Links  big screw_v1 (Autodesk Fusion 360 design; units mm, degrees)
Autodesk Fusion 360 part; units mm, degrees
note: some values were not read from the file. Chosen so that the rebuilt part matches the saved one: which bodies a step acts on. Set by a fixed rule: which sketch regions a step uses.
sketch "passive link sketch" plane through (0, 0, 0) normal (0, 0, 1) x (1, 0, 0)
  line L0 (-18.5, 6) -> (-18.5, -6) construction
  line L1 (18.5, -6) -> (18.5, 6) construction
  line L2 (18.5, 6) -> (-18.5, -6) construction
  line L3 (-18.5, 6) -> (18.5, -6) construction
  circle A0 centre (12.5, 0) radius 4
  circle A1 centre (12.5, 0) radius 2.975
  circle A2 centre (12.5, 0) radius 6
  line L4 (0, 6) -> (0, -15) construction
  line L5 (12.5, 6) -> (0, 6)
  line L6 (0, -6) -> (12.5, -6)
  line L7 (12.5, -6) -> (12.5, 6)
  line L8 (12.5, 6) -> (-12.5, -6) construction
  line L9 (-12.5, 6) -> (12.5, -6) construction
  line L10 (18.5, 6) -> (0, 6) construction
  line L11 (-12.5, 6) -> (-18.5, 6) construction
  line L12 (-18.5, -6) -> (-12.5, -6) construction
  line L13 (0, -6) -> (18.5, -6) construction
  line L14 (0, -6) -> (-18.5, -6) construction
  line L15 (-12.5, -6) -> (-12.5, 6)
  line L16 (-18.5, 6) -> (0, 6) construction
  circle A3 centre (-12.5, 0) radius 6
  circle A4 centre (-12.5, 0) radius 2.975
  circle A5 centre (-12.5, 0) radius 4
  line L17 (0, -6) -> (-12.5, -6)
  line L18 (-12.5, 6) -> (0, 6)
  dimension "d2" = 12
  dimension "d3" = 8
  dimension "d4" = 5.95
  dimension "d5" = 12
  dimension "d6" = 12.5
  dimension "d7" = 25
  constraint horizontal L10
  constraint perpendicular L0 L10
  constraint parallel L10 L12
  constraint parallel L0 L1
  constraint coincident L2 origin
  constraint coincident L3 origin
  constraint concentric A0 A1
  constraint concentric A0 A2
  constraint perpendicular L4 L12
  constraint horizontal origin A0.centre
  constraint horizontal L5
  constraint parallel L5 L6
  constraint coincident A2 L5.start
  constraint coincident L8 origin
  constraint coincident L9 origin
  constraint collinear L10 L11
  constraint coincident L4 L6.start
  constraint collinear L12 L13
  constraint symmetric L1.end L4 L0.start
  constraint symmetric L1.start L4 L0.end
  constraint symmetric A0 L4 A5
  constraint symmetric A1 L4 A4
  constraint symmetric A2 L4 A3
  constraint symmetric L4 L5.start L9.start
  constraint symmetric L4 L6.end L8.end
  constraint symmetric L4 L5.end L10.end
  constraint symmetric L4 L6.start L13.start
  constraint perpendicular L15 L18
  measures "d2" distance of L0.start L0.end
  measures "d3" diameter of A0
  measures "d4" diameter of A1
  measures "d5" diameter of A2
  measures "d6" distance of origin A0.centre
  measures "d7" distance of L8.end L6.end
extrude "base" add sketch "passive link sketch" along normal mid plane 4 contours A2 L5 L6 A3 L17 L18 makes body 1
extrude "l  big cyl" add sketch "passive link sketch" along normal blind 3 and the other way blind 7 separate body contours L15 A3 A5 | L15 A3 A5 | L15 A4 A5 | L15 A4 A5 makes body 2
fillet "Fillet6" radius 1 1 edges at (-18.094, -2.1697, 3) on bodies 2
extrude "Extrude8" add sketch "passive link sketch" along normal blind 4 and the other way blind 7 separate body contours L15 A4 A5 | L15 A4 A5 makes body 3
sketch "Square nut hole" plane through (0, 0, -7) normal (0, 0, -1) x (1, 0, 0)
  circle A0 centre (-12.5, 0) radius 2.975
  circle A1 centre (-12.5, 0) radius 4
  line L0 (-15.6, 3.1) -> (-9.4, 3.1)
  line L1 (-9.4, 3.1) -> (-9.4, -3.1)
  line L2 (-9.4, -3.1) -> (-15.6, -3.1)
  line L3 (-15.6, -3.1) -> (-15.6, 3.1)
  line L4 (-15.6, 3.1) -> (-9.4, -3.1) construction
  line L5 (-9.4, 3.1) -> (-15.6, -3.1) construction
  point P0 (-12.5, 0)
  dimension "d132" = 6.2
  dimension "d133" = 6.2
  constraint horizontal L0
  constraint perpendicular L0 L1
  constraint parallel L0 L2
  constraint parallel L1 L3
  constraint coincident L4 P0
  constraint coincident L5 P0
  constraint coincident P0 A0.centre
  measures "d132" distance of L1.end L2.end
  measures "d133" distance of L0.end L1.end
extrude "Extrude17" cut sketch "Square nut hole" against normal blind 3.5 contours A0 | A1 L0 L1 L2 L3 | A1 L0 L1 | A1 L1 L2 | A1 L0 L3 | A1 L2 L3 bodies 2 3
mirror "Mirror1" about plane through (0, 0, 0) normal (1, 0, 0) of bodies 1 2 3 makes body 4 at (6.5075, -0.2991, -4) makes body 5 at (12.5, 4, 0.3333) makes body 6 at (-2.1723, -0.1495, 2)
mirror "Mirror2" about plane through (0, 0, 0) normal (0, 0, 1) of bodies 4 5 makes body 7 at (6.5075, -0.2991, 4) makes body 8 at (12.5, 4, -0.3333)
delete_body "RemoveBody1" bodies 4
delete_body "RemoveBody2" bodies 5
sketch "motorLinkSketch" plane through (0, 0, 0) normal (0, 0, 1) x (1, 0, 0) in component "MotorLinkComponent"
  circle A0 centre (-12.5, 0) radius 1
  line L0 (18.5, 6) -> (-18.5, -6) construction
  circle A1 centre (-12.5, 0) radius 2.975
  line L1 (-12.5, 6) -> (-18.5, 6) construction
  line L2 (-18.5, -6) -> (-12.5, -6) construction
  circle A2 centre (12.5, 0) radius 1
  line L3 (0, -6) -> (-12.5, -6)
  line L4 (-12.5, -6) -> (-12.5, 6)
  line L5 (-12.5, 6) -> (0, 6)
  line L6 (14.65, -1.462) -> (14.65, 1.462)
  line L7 (12.5, 6) -> (0, 6)
  line L8 (18.5, 6) -> (0, 6) construction
  line L9 (0, -6) -> (12.5, -6)
  line L10 (-18.5, 6) -> (-18.5, -6) construction
  line L11 (0, 6) -> (0, -15) construction
  line L12 (18.5, -6) -> (18.5, 6) construction
  line L13 (-18.5, 6) -> (0, 6) construction
  line L14 (0, -6) -> (18.5, -6) construction
  circle A3 centre (12.5, 0) radius 2.6
  circle A4 centre (-12.5, 0) radius 6
  line L15 (0, -6) -> (-18.5, -6) construction
  line L16 (-18.5, 6) -> (18.5, -6) construction
  line L17 (12.5, 6) -> (-12.5, -6) construction
  line L18 (12.5, -6) -> (12.5, 6)
  circle A5 centre (12.5, 0) radius 6
  line L19 (-12.5, 6) -> (12.5, -6) construction
  dimension "d65" = 12
  dimension "d66" = 2
  dimension "d67" = 5.2
  dimension "d68" = 12
  dimension "d69" = 12.5
  dimension "d70" = 25
  dimension "d71" = 2.15
  dimension "d72" = 5.95
  constraint horizontal L8
  constraint perpendicular L8 L10
  constraint parallel L2 L8
  constraint parallel L10 L12
  constraint coincident origin L0
  constraint coincident origin L16
  constraint concentric A2 A3
  constraint concentric A2 A5
  constraint perpendicular L2 L11
  constraint horizontal A2.centre origin
  constraint horizontal L7
  constraint parallel L7 L9
  constraint coincident L7.start A5
  constraint coincident origin L17
  constraint coincident origin L19
  constraint collinear L1 L8
  constraint coincident L3.start L11
  constraint collinear L2 L14
  constraint symmetric L1.end L0.start L11
  constraint symmetric L0.end L12.start L11
  constraint symmetric A0 A2 L11
  constraint symmetric L11 A4 A5
  constraint symmetric L7.start L1.start L11
  constraint symmetric L9.end L2.end L11
  constraint symmetric L5.end L7.end L11
  constraint symmetric L3.start L9.start L11
  constraint perpendicular L4 L5
  constraint coincident L6.start A3
  constraint coincident L6.end A3
  constraint vertical L6
  measures "d65" distance of L1.end L0.end
  measures "d66" diameter of A2
  measures "d67" diameter of A3
  measures "d68" diameter of A5
  measures "d69" distance of A2.centre origin
  measures "d70" distance of L9.end L2.end
  measures "d71" distance of A2.centre L6
  measures "d72" diameter of A1
extrude "Extrude5" [suppressed] in component "MotorLinkComponent"
extrude "Extrude3" [suppressed] in component "MotorLinkComponent"
extrude "Extrude4" [suppressed] in component "MotorLinkComponent"
extrude "Extrude12" [suppressed]
fillet "Fillet1" [suppressed] in component "MotorLinkComponent"
extrude "Extrude2" [suppressed] in component "MotorLinkComponent"
extrude "Extrude1" [suppressed] in component "MotorLinkComponent"
fillet "Fillet2" [suppressed] in component "MotorLinkComponent"
sketch "top nut" plane through (0, 0, 5) normal (0, 0, 1) x (-1, 0, 0) in component "MotorLinkComponent"
  circle A0 centre (12.5, 0) radius 1
  circle A1 centre (12.5, 0) radius 2.975
  line L0 (14.5842, -1.3806) -> (14.7377, 1.1147)
  line L1 (12.3465, -2.4953) -> (14.5842, -1.3806)
  line L2 (10.2623, -1.1147) -> (12.3465, -2.4953)
  circle A2 centre (12.5, 0) radius 1
  circle A3 centre (12.5, 0) radius 2.5 construction
  line L3 (12.6535, 2.4953) -> (10.4158, 1.3806)
  arc A4 (12.5, -6) -> (12.5, 6) centre (12.5, 0) ccw
  line L4 (10.4158, 1.3806) -> (10.2623, -1.1147)
  line L5 (14.7377, 1.1147) -> (12.6535, 2.4953)
  point P0 (12.5, 0)
  dimension "d106" = 5
  constraint coincident P0 A0.centre
  constraint coincident L0.start A3
  measures "d106" diameter of A3
extrude "Extrude6" [suppressed] in component "MotorLinkComponent"
sketch "spacer" plane through (0, 0, 0) normal (0, 0, 1) x (1, 0, 0)
  circle A0 centre (-61, 0) radius 4
  circle A1 centre (-61, 0) radius 1
  dimension "d123" = 8
  dimension "d126" = 2
  constraint concentric A0 A1
  measures "d123" diameter of A0
  measures "d126" diameter of A1
extrude "Extrude16" [suppressed]
hole "Hole1" [suppressed] in component "MotorLinkComponent"
equation "d2 = BigBarrelDiam"
equation "d4 = nipDiameter"
equation "d5 = BigBarrelDiam"
equation "d25 = 0.0 °"
equation "d53 = 0.0 °"
equation "rect = 10 mm"
equation "shoulder = 2 mm"
equation "regularNip = 5 mm"
equation "hex = 4 mm"
equation "nipDiameter = 5.95 mm"
equation "BigBarrelDiam = 12 mm"
equation "smallerHoleDiam = 2 mm"
equation "d66 = smallerHoleDiam"
equation "d67 = motorShaftDiameter"
equation "d68 = BigBarrelDiam"
equation "d72 = nipDiameter"
equation "motorShaftDiameter = 5.2 mm"
equation "d76 = rect / 2"
equation "d80 = rect / 2 + shaftNip"
equation "d82 = rect / 2"
equation "d83 = 0.0 °"
equation "d84 = rect / 2 + shaftNip"
equation "d86 = rect / 2"
equation "d87 = 0.0 °"
equation "d88 = rect / 2"
equation "d90 = rect / 2 + shoulder"
equation "d91 = 0.0 °"
equation "d92 = rect / 2"
equation "d94 = rect / 2 + shoulder + regularNip"
equation "d95 = 0.0 °"
equation "shaftNip = 5.9 mm"
equation "rectLen = 25 mm"
equation "d98 = rect / 2"
equation "d100 = rect / 2"
equation "d101 = 0.0 °"
equation "d109 = rect / 2"
equation "d111 = rect / 2 + shoulder + regularNip"
equation "d112 = 0.0 °"
equation "d113 = rect / 2 + shoulder + regularNip"
equation "d114 = 0.0 °"
named bodies: "PassiveLinkRectangleBody", "big barrel motor shaft", "big barrel", "nip", "rect", "spacer", "screwHole", "big barrel (1)", "screwHole (1)", "big barrel (1) (1)", "screwHole (1) (1)", "PassiveLinkRectangleBody (1)"
